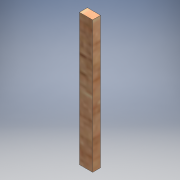
# Autodesk Inventor part: LevelingBar
Saved by Autodesk Inventor 2016 (Build 200138000, 138)
## iProperties
Created: 2016-04-01
Part Number: LevelingBar
Material: Wood (Birch)
Document SubType Name: Modeling
Designer: mkepler
Mass: 0.4125 g
Surface Area: 8.3 cm^2
Volume: 0.75 cm^3
Density: 0.55 g/cm^3
Appearance: Birch - Natural Polished
Author: mkepler
Autodesk Inventor part; units mm, degrees
ref_plane "YZ Plane" through (0, 0, 0) normal (1, 0, 0) x (0, 1, 0)
ref_plane "XZ Plane" through (0, 0, 0) normal (0, 1, 0) x (-1, 0, 0)
ref_plane "XY Plane" through (0, 0, 0) normal (0, 0, 1) x (1, 0, 0)
sketch "Sketch1" plane through (0, 0, 0) normal (0, 1, 0) x (-1, 0, 0)
  line L0 (0, 0) -> (5, 0)
  line L1 (5, 0) -> (5, -50)
  line L2 (5, -50) -> (0, -50)
  line L3 (0, -50) -> (0, 0)
  dimension "d0" = 5
  dimension "d1" = 50
  constraints: 8 end point, 2 parallel, 1 horizontal, 1 perpendicular
  measures "d0" distance of L1.end L2.end
  measures "d1" distance of L0.end L1.end
extrude "Extrusion1" add sketch "Sketch1" along normal blind 3
body "Solid1"
